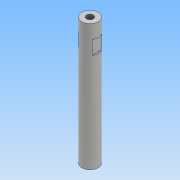
# Autodesk Inventor part: Top_Separator Weight
Saved by Autodesk Inventor 2018.1 (Build 221171000, 171)
## iProperties
Created: 2019-02-11
Part Number: Top_Separator Weight
Material: Aluminum 6061
Document SubType Name: Modeling
Designer: James
Density: 2.7 g/cm^3
Appearance: Aluminum - Flat
Author: James
Autodesk Inventor part; units mm, degrees
ref_plane "YZ Plane" through (0, 0, 0) normal (1, 0, 0) x (0, 1, 0)
ref_plane "XZ Plane" through (0, 0, 0) normal (0, 1, 0) x (-1, 0, 0)
ref_plane "XY Plane" through (0, 0, 0) normal (0, 0, 1) x (1, 0, 0)
sketch "Sketch1" plane through (0, 0, 0) normal (0, 0, 1) x (1, 0, 0)
  circle A0 centre (0, 0) radius 3
  dimension "d0" = 6
  constraints: 1 centre point, 1 coincident
  measures "d0" diameter of A0
extrude "Extrusion1" add sketch "Sketch1" along normal mid plane 46
sketch "Sketch2" plane through (0, 0, 23) normal (0, 0, 1) x (1, 0, 0)
  point P0 (0, 0)
  point P1 (0, 0)
  constraints: 1 coincident
hole "Hole1" at (0, 0, 23) direction (0, 0, -1) diameter 2.459 depth 8.8 tip angle 118 thread size "M3x0.5" class "6H" standard "ANSI Metric M Profile"
sketch "Sketch3" plane through (0, 0, 0) normal (0, 1, 0) x (-1, 0, 0)
  line L0 (3, -23) -> (3, 23) projected
  line L1 (3, 18) -> (2.5, 18)
  line L2 (2.5, 18) -> (2.5, 13)
  line L3 (2.5, 13) -> (3, 13)
  line L4 (3, 13) -> (3, 18)
  line L5 (-3, 18) -> (-2.5, 18)
  line L6 (-2.5, 18) -> (-2.5, 13)
  line L7 (-2.5, 13) -> (-3, 13)
  line L8 (-3, 13) -> (-3, 18)
  line L9 (3, 23) -> (-3, 23) projected
  point P0 (0, 0)
  dimension "d10" = 0.5
  dimension "d11" = 5
  dimension "d12" = 0.5
  dimension "d16" = 5
  dimension "d19" = 5
  dimension "d20" = 6
  dimension "d21" = 6
  constraints: 16 end point, 4 parallel, 2 horizontal, 2 horizontal alignment, 2 perpendicular, 2 point on line
  measures "d10" distance between parallel lines of L0 L2
  measures "d11" distance between parallel lines of L6 L2
  measures "d12" distance between parallel lines of L6 L8
  measures "d16" distance of L7.end L5.start
  measures "d19" distance between parallel lines of L9 L5
  measures "d20" distance between parallel lines of L0 L8
  measures "d21" distance of L0.end L9.end
extrude "Extrusion2" cut sketch "Sketch3" along normal through all both and the other way through all
mirror "Mirror1" about plane through (0, 0, 0) normal (0, 0, 1) of "Hole1"
equation "\"d10\" = d12"
equation "\"d20\" = d21"
body "Solid1"
